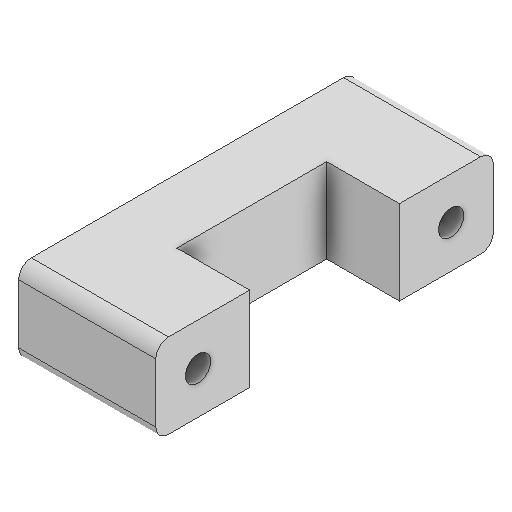
# Autodesk Inventor part: 3DP_ASA_Balcony_Mounting_Clamp_Back
Saved by Autodesk Inventor 2026.1 (Build 301233000, 233)
## iProperties
Created: 2025-06-22
Part Number: 3DP_ASA_Balcony_Mounting_Clamp_Back
Material: Generic
Document SubType Name: Modeling
Designer: User
Density: 1 g/cm^3
Appearance: Default
Author: User
Autodesk Inventor part; units mm, degrees
ref_plane "YZ Plane" through (0, 0, 0) normal (1, 0, 0) x (0, 1, 0)
ref_plane "XZ Plane" through (0, 0, 0) normal (0, 1, 0) x (-1, 0, 0)
ref_plane "XY Plane" through (0, 0, 0) normal (0, 0, 1) x (1, 0, 0)
sketch "Sketch1" plane through (0, 0, 0) normal (0, 1, 0) x (-1, 0, 0)
  line L0 (-16.25, 40) -> (16.25, 40)
  line L1 (16.25, 40) -> (16.25, -40)
  line L2 (16.25, -40) -> (-16.25, -40)
  line L3 (-16.25, -40) -> (-16.25, 40)
  point P0 (0, 0)
  dimension "d0" = 80
  dimension "d1" = 32.5
  dimension "d2" = 40
  dimension "d3" = 16.25
  constraints: 8 end point, 2 parallel, 1 horizontal, 1 perpendicular
  measures "d0" distance between parallel lines of L2 L0
  measures "d1" distance between parallel lines of L3 L1
  measures "d2" distance from line of point (0, 0) L0
  measures "d3" distance from line of L1 point (0, 0)
extrude "Extrusion1" add sketch "Sketch1" along normal blind 20
sketch "Sketch2" plane through (16.25, 0, 40) normal (1, 0, 0) x (0, 0, -1)
  line L0 (0, 0) -> (80, 0) projected
  line L1 (80, 0) -> (80, 20) projected
  line L2 (0, 20) -> (80, 20) projected
  line L3 (0, 0) -> (0, 20) projected
  point P0 (40, 0)
  point P1 (10, 10)
  point P2 (70, 10)
  dimension "d8" = 10
  dimension "d9" = 10
  dimension "d10" = 10
  dimension "d11" = 10
  measures "d8" distance from line of L3 point (10, 10)
  measures "d9" distance from line of L1 point (70, 10)
  measures "d10" distance from line of L2 point (10, 10)
  measures "d11" distance from line of L2 point (70, 10)
hole "Hole1" at (16.25, 10, 30) at (16.25, 10, -30) direction (-1, 0, 0) diameter 6 end through all
sketch "Sketch3" plane through (0, 20, 0) normal (0, 1, 0) x (1, 0, 0)
  line L0 (16.25, -40) -> (16.25, 40) projected
  line L1 (16.25, 40) -> (-16.25, 40) projected
  line L2 (-16.25, 40) -> (-16.25, -40) projected
  line L3 (-16.25, -40) -> (16.25, -40) projected
  line L4 (16.25, -17.75) -> (-1, -17.75)
  line L5 (-1, -17.75) -> (-1, 17.75)
  line L6 (-1, 17.75) -> (16.25, 17.75)
  point P0 (0, 0)
  dimension "d19" = 17.25
  dimension "d20" = 35.5
  dimension "d21" = 17.75
  constraints: 6 end point, 2 perpendicular, 2 point on line, 1 horizontal
  measures "d19" distance between parallel lines of L0 L5
  measures "d20" distance between parallel lines of L6 L4
  measures "d21" distance from line of point (0, 0) L4
extrude "Extrusion2" cut sketch "Sketch3" against normal through all contours L4 L5 L6 L0
fillet "Fillet1" radius 3 4 edges at (0, 20, 40) (0, 0, 40) (0, 20, -40) (0, 0, -40)
equation "\"d2\" = 0.5 * d0"
equation "\"d3\" = 0.5 * d1"
equation "\"d9\" = d8"
equation "\"d21\" = 0.5 * d20"
body "Solid1"
